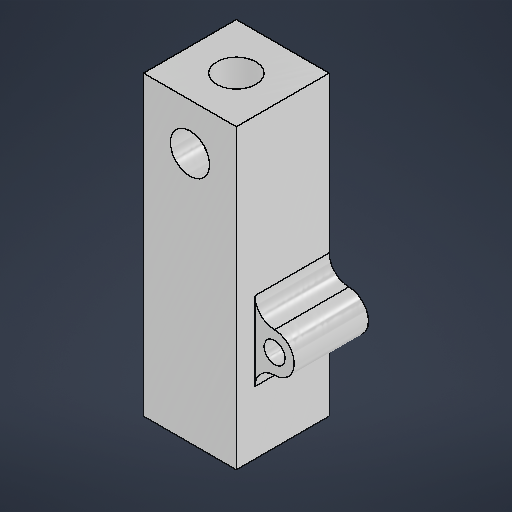
# Autodesk Inventor part: A Idler
Saved by Autodesk Inventor 2026 (Build 300175050, 175E)
## iProperties
Created: 2025-04-15
Part Number: A Idler
Material: Aluminum 6061
Document SubType Name: Modeling
Designer: Joshua Eah
Density: 2.7 g/cm^3
Appearance: Machined - Aluminum
Author: Joshua Eah
Autodesk Inventor part; units mm, degrees
ref_plane "YZ Plane" through (0, 0, 0) normal (1, 0, 0) x (0, 1, 0)
ref_plane "XZ Plane" through (0, 0, 0) normal (0, 1, 0) x (-1, 0, 0)
ref_plane "XY Plane" through (0, 0, 0) normal (0, 0, 1) x (1, 0, 0)
sketch "Base Profile" plane through (0, 0, 0) normal (0, 1, 0) x (-1, 0, 0)
  line L0 (0, 0) -> (15, 0)
  line L1 (15, 0) -> (15, -15)
  line L2 (15, -15) -> (0, -15)
  line L3 (0, -15) -> (0, 0)
  line L4 (15, -15) -> (15, 0)
  line L5 (15, -15) -> (0, -15)
  line L6 (0, -15) -> (0, -21.35)
  line L7 (0, -21.35) -> (15, -21.35)
  line L8 (15, -21.35) -> (15, -15)
  dimension "d164" = 15
  dimension "d165" = 15
  dimension "d360" = 6.35
  constraints: 18 end point, 5 point on line, 4 parallel, 2 horizontal, 2 perpendicular
  measures "d164" distance of L1.end L2.end
  measures "d165" distance of L0.end L1.end
  measures "d360" distance of L7.end L4.start
extrude "Stock" add sketch "Base Profile" against normal blind 33
extrude "Extrusion Post" add sketch "Base Profile" along normal blind 15 contours L0 L1 L2 L3
sketch "Front Pattern" plane through (0, -33, -21.35) normal (1, 0, 0) x (0, 0, -1)
  line L0 (-21.35, 0) -> (-21.35, 48) projected
  line L1 (0, 0) -> (-21.35, 0) projected
  line L2 (0, 33) -> (0, 0) projected
  line L3 (-6.35, 33) -> (0, 33) projected
  line L4 (-6.35, 33) -> (-6.35, 48) projected
  line L5 (-21.35, 48) -> (-6.35, 48) projected
  circle A0 centre (-13.85, 40.5) radius 3.175
  line L6 (-6.35, 33) -> (-6.35, 0)
  line L7 (-6.35, 16.5) -> (0, 16.5)
  circle A1 centre (-3.175, 16.5) radius 1.5
  line L8 (-6.35, 19.675) -> (0, 19.675)
  line L9 (0, 19.675) -> (0, 13.325)
  line L10 (0, 13.325) -> (-6.35, 13.325)
  line L11 (-6.35, 13.325) -> (-6.35, 19.675)
  line L12 (-6.35, 19.675) -> (0, 13.325) construction
  line L13 (0, 19.675) -> (-6.35, 13.325) construction
  point P0 (-6.35, 13.325)
  point P1 (-6.35, 19.675)
  dimension "d361" = 6.35
  dimension "d362" = 7.5
  dimension "d363" = 7.5
  dimension "d364" = 3
  dimension "d365" = 6.35
  constraints: 16 end point, 5 midpoint, 2 centre point, 2 parallel, 2 perpendicular, 2 point on line, 1 horizontal
  measures "d361" diameter of A0
  measures "d362" distance from line of A0.centre L0
  measures "d363" distance from line of A0.centre L5
  measures "d364" diameter of A1
  measures "d365" distance between parallel lines of L10 L8
extrude "Extrusion19" cut sketch "Front Pattern" against normal through all contours L6 L10 L2 L1 | L3 L2 L8 L6
extrude "Extrusion20" cut sketch "Front Pattern" against normal blind 3 contours L6 L7 A1 L2 L10 | L6 L8 L2 L7 A1 | A1 L7 | L7 A1
hole "Hole24" at (0, 7.5, -7.5) direction (-1, 0, 0) diameter 3.4036 end through all start extended yes counterbore diameter 6.35 counterbore depth 13 clearance for "Socket Head Cap Screw" size "M3" standard "Ansi Metric M Profile"
hole "Hole23" at (0, -16.5, -18.175) direction (-1, 0, 0) diameter 3.4036 end through all start extended yes clearance for "Flat Head Machine Screw" size "M3" standard "Ansi Metric M Profile"
fillet "Fillet3" radius 3.175 4 edges at (-9, -13.325, -21.35) (-9, -19.675, -21.35) (-9, -13.325, -15) (-9, -19.675, -15)
sketch "Sketch36" plane through (0, 15, 0) normal (0, 1, 0) x (1, 0, 0)
  line L0 (-15, 15) -> (-15, 0) projected
  line L1 (-15, 0) -> (0, 0) projected
  line L2 (0, 0) -> (0, 15) projected
  line L3 (0, 15) -> (-15, 15) projected
  circle A0 centre (-7.5, 7.5) radius 3.175
  dimension "d385" = 6.35
  dimension "d386" = 7.5
  dimension "d387" = 7.5
  constraints: 1 centre point
  measures "d385" diameter of A0
  measures "d386" distance from line of A0.centre L1
  measures "d387" distance from line of A0.centre L0
hole "Hole25" at (-7.5, 15, -7.5) direction (0, -1, 0) diameter 3.4036 end through all start extended yes counterbore diameter 6.35 counterbore depth 12.675 clearance for "Socket Head Cap Screw" size "M3" standard "Ansi Metric M Profile"
sketch "Left Pattern" plane through (-15, -33, 0) normal (0, 0, 1) x (1, 0, 0)
  line L0 (0, 0) -> (0, 48) projected
  line L1 (15, 0) -> (0, 0) projected
  line L2 (15, 0) -> (15, 48) projected
  line L3 (0, 48) -> (15, 48) projected
  circle A0 centre (7.5, 40.5) radius 1.5
  circle A1 centre (7.5, 7.5) radius 1.5
  dimension "d395" = 3
  dimension "d396" = 7.5
  dimension "d397" = 7.5
  dimension "d398" = 3
  dimension "d399" = 7.5
  constraints: 2 centre point, 1 vertical alignment
  measures "d395" diameter of A0
  measures "d396" distance from line of L3 A0.centre
  measures "d397" distance from line of A0.centre L2
  measures "d398" diameter of A1
  measures "d399" distance from line of L1 A1.centre
hole "Hole26" at (-7.5, 7.5, 0) at (-7.5, -25.5, 0) direction (0, 0, -1) diameter 2.459 end up to face face through (-7.5, -39.6335, -7.5) facing (0, 1, 0) round with radius 1.7018 far side no start extended yes thread size "M3x0.5" class "6H" standard "ANSI Metric M Profile"
equation "\"d164\" = extrusionWidth"
equation "\"d168\" = extrusionOffset"
equation "\"extrusionWidth\" = 15"
equation "\"idlerLength\" = 18"
equation "\"bearingOffsetFromBottom\" = 7.5"
equation "\"extrusionOffset\" = 33"
equation "\"bearingStackHeight\" = 9"
equation "\"bearingSlotLength\" = 5"
equation "\"bearingClearance\" = 13"
equation "\"pinSupportLength\" = 2"
body "Solid2"
